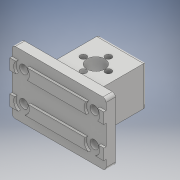
# Autodesk Inventor part: CarroZ - EixoZ
Saved by Autodesk Inventor 2017 (Build 210142000, 142)
## iProperties
Created: 2020-08-03
Part Number: CarroZ - EixoZ
Material: Generic
Document SubType Name: Modeling
Designer: ale
Density: 1 g/cm^3
Appearance: Default
Author: ale
Autodesk Inventor part; units mm, degrees
ref_plane "YZ Plane" through (0, 0, 0) normal (1, 0, 0) x (0, 1, 0)
ref_plane "XZ Plane" through (0, 0, 0) normal (0, 1, 0) x (-1, 0, 0)
ref_plane "XY Plane" through (0, 0, 0) normal (0, 0, 1) x (1, 0, 0)
sketch "Sketch1" plane through (0, 0, 0) normal (0, 0, 1) x (1, 0, 0)
  circle A0 centre (0, 0) radius 5.75
  circle A1 centre (0, 8) radius 2
  circle A2 centre (8, 0) radius 2
  circle A3 centre (0, -8) radius 2
  circle A4 centre (-8, 0) radius 2
  line L0 (-15, 17.5) -> (15, 17.5)
  line L1 (15, 17.5) -> (15, -17.5)
  line L2 (15, -17.5) -> (-15, -17.5)
  line L3 (-15, -17.5) -> (-15, 17.5)
  line L4 (-15, 17.5) -> (15, -17.5) construction
  line L5 (15, 17.5) -> (-15, -17.5) construction
  dimension "d0" = 11.5
  dimension "d2" = 4
  dimension "d3" = 4
  dimension "d4" = 4
  dimension "d5" = 4
  dimension "d6" = 30
  dimension "d7" = 35
  constraints: 12 end point, 5 centre point, 2 midpoint, 2 parallel, 1 coincident, 1 horizontal, 1 perpendicular
  measures "d0" diameter of A0
  measures "d2" diameter of A1
  measures "d3" diameter of A2
  measures "d4" diameter of A3
  measures "d5" diameter of A4
  measures "d6" distance of L1.end L2.end
  measures "d7" distance of L0.end L1.end
extrude "Extrusion1" add sketch "Sketch1" along normal blind 25
sketch "Sketch2" plane through (-15, -17.5, 0) normal (0, -1, 0) x (1, 0, 0)
  line L0 (0, 0) -> (0, 25) projected
  line L1 (30, 0) -> (0, 0) projected
  line L2 (0, 25) -> (30, 0)
  line L3 (-15, 32.5) -> (45, 32.5)
  line L4 (45, 32.5) -> (45, -7.5)
  line L5 (45, -7.5) -> (-15, -7.5)
  line L6 (-15, -7.5) -> (-15, 32.5)
  line L7 (-15, 32.5) -> (45, -7.5) construction
  line L8 (45, 32.5) -> (-15, -7.5) construction
  point P0 (15, 0)
  point P1 (15, 12.5)
  dimension "d10" = 60
  dimension "d11" = 40
  constraints: 14 end point, 3 midpoint, 2 parallel, 1 horizontal, 1 perpendicular
  measures "d10" distance of L4.end L5.end
  measures "d11" distance of L3.end L4.end
extrude "Extrusion2" add sketch "Sketch2" along normal blind 6 contours L0 L2 L1 | L3 L4 L5 L6
sketch "Sketch3" plane through (-15, -23.5, 0) normal (0, -1, 0) x (1, 0, 0)
  line L0 (-15, -7.5) -> (-15, 32.5) projected
  line L1 (45, 32.5) -> (45, -7.5) projected
  line L2 (-15, 26) -> (45, 26)
  line L3 (-15, 19) -> (45, 19)
  line L4 (-15, 6) -> (45, 6)
  line L5 (-15, -1) -> (45, -1)
  line L6 (45, 26) -> (45, 19)
  line L7 (45, 6) -> (45, -1)
  line L8 (-15, -1) -> (-15, 6)
  line L9 (-15, 19) -> (-15, 26)
  point P0 (15, 0)
  constraints: 16 end point, 4 perpendicular
extrude "Extrusion3" add sketch "Sketch3" along normal blind 1.5 contours L0 L4 L1 L5 | L0 L2 L1 L3
sketch "Sketch4" plane through (-15, -25, 0) normal (0, -1, 0) x (1, 0, 0)
  line L0 (-15, 26) -> (45, 26) projected
  line L1 (45, 26) -> (30, 19)
  line L2 (-15, 19) -> (45, 19) projected
  line L3 (30, 0) -> (30, 25) projected
  line L4 (30, 13) -> (5, 13)
  line L5 (5, 0) -> (5, 25) projected
  line L6 (45, -7.5) -> (-15, -7.5) projected
  line L7 (15, -7.5) -> (15, 32.5)
  line L8 (45, 32.5) -> (-15, 32.5) projected
  point P0 (15, 0)
  point P1 (37.5, 22.5)
  point P2 (37.5, 3.5)
  point P3 (-7.5, 22.5)
  point P4 (-7.5, 3.5)
  constraints: 6 end point, 4 point on line, 3 midpoint, 3 symmetric about line
hole "Hole1" at (22.5, -25, 22.5) at (22.5, -25, 3.5) at (-22.5, -25, 22.5) at (-22.5, -25, 3.5) direction (0, 1, 0) diameter 5.5 end through all counterbore diameter 10 counterbore depth 1.5
fillet "Fillet1" radius 2 8 edges at (15, 17.5, 12.5) (0, 17.5, 25) (-15, 17.5, 12.5) (0, 17.5, 0) (-30, -20.5, -7.5) (30, -20.5, -7.5) (30, -20.5, 32.5) (-30, -20.5, 32.5)
body "Solid1"
